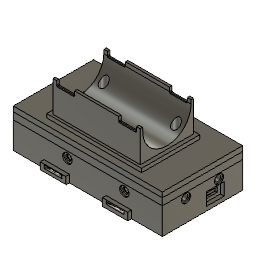
Display (Autodesk Fusion 360 design; units mm, degrees)
Autodesk Fusion 360 part; units mm, degrees
sketch "Sketch1" plane through (0, 0, 0) normal (0, 0, 1) x (1, 0, 0)
  line L0 (20.6, 4.75) -> (97.2, 4.75)
  line L1 (97.2, 4.75) -> (97.2, 56.75)
  line L2 (97.2, 56.75) -> (20.6, 56.75)
  line L3 (20.6, 56.75) -> (20.6, 4.75)
  line L4 (0, 0) -> (117.8, 0)
  line L5 (117.8, 0) -> (117.8, 63.5)
  line L6 (117.8, 63.5) -> (0, 63.5)
  line L7 (0, 63.5) -> (0, 0)
  dimension "d1" = 76.6
  dimension "d2" = 52
  dimension "d4" = 64
  dimension "d5" = 4.75
  dimension "d6" = 20.6
  dimension "d41" = 20.6
  dimension "d47" = 6.75
  constraint horizontal L0
  constraint vertical L1
  constraint horizontal L2
  constraint vertical L3
  constraint horizontal L4
  constraint vertical L5
  constraint horizontal L6
  constraint vertical L7
  constraint coincident L4.start L7.end
  measures "d1" distance of L0.start L0.end
  measures "d2" distance of L0.start L2.end
  measures "d5" distance of L0 L4
  measures "d6" distance of L3 L7
  measures "d41" distance of L1 L5
  measures "d47" distance of L2 L6
extrude "Extrude1" add sketch "Sketch1" along normal blind 1 makes body 1
sketch "Sketch2" plane through (0, 0, 1) normal (0, 0, 1) x (-1, 0, 0)
  line L0 (-20.6, -4.75) -> (-20.6, -56.75)
  line L1 (-20.6, -56.75) -> (-97.2, -56.75)
  line L2 (-97.2, -56.75) -> (-97.2, -4.75)
  line L3 (-97.2, -4.75) -> (-20.6, -4.75)
  line L4 (0, -63.5) -> (0, 0)
  line L5 (0, 0) -> (-117.8, 0)
  line L6 (-117.8, 0) -> (-117.8, -63.5)
  line L7 (-117.8, -63.5) -> (0, -63.5)
  line L8 (-18.6, -58.5) -> (-105.6, -58.5)
  line L9 (-105.6, -58.5) -> (-105.6, -3)
  line L10 (-105.6, -3) -> (-18.6, -3)
  line L11 (-18.6, -3) -> (-18.6, -58.5)
  dimension "d9" = 55.5
  dimension "d14" = 2
  dimension "d15" = 8.4
  dimension "d46" = 1.75
  constraint horizontal L8
  constraint vertical L9
  constraint horizontal L10
  constraint vertical L11
  measures "d9" distance of L8.start L10.end
  measures "d14" distance of L0 L11
  measures "d15" distance of L2 L9
  measures "d46" distance of L1 L8
extrude "Extrude2" add sketch "Sketch2" along normal blind 4.56 contours L4 L5 L6 L7 bodies 1
sketch "Sketch3" plane through (0, 0, 5.56) normal (0, 0, 1) x (-1, 0, 0)
  line L0 (-18.6, -3) -> (-18.6, -58.5)
  line L1 (-18.6, -58.5) -> (-105.6, -58.5)
  line L2 (-105.6, -58.5) -> (-105.6, -3)
  line L3 (-117.8, -63.5) -> (0, -63.5)
  line L4 (0, -63.5) -> (0, 0)
  line L5 (0, 0) -> (-117.8, 0)
  line L6 (-117.8, 0) -> (-117.8, -63.5)
  line L7 (-11, -50.1) -> (-18.1, -50.1)
  line L8 (-18.1, -50.1) -> (-18.1, -43.1)
  line L9 (-18.1, -43.1) -> (-11, -43.1)
  line L10 (-11, -43.1) -> (-11, -50.1)
  circle A0 centre (-14.3, -54.9) radius 1.35
  line L11 (-9.2, -61.5) -> (-113, -61.5)
  line L12 (-113, -2) -> (-9.2, -2)
  line L13 (-9.2, -2) -> (-9.2, -61.5)
  line L14 (-105.6, -3) -> (-18.6, -3)
  circle A1 centre (-14.5, -6.6) radius 1.35
  line L15 (-14.5, -66.6204) -> (-14.5, 2.7727) construction
  line L16 (4.0638, -54.9) -> (-136.0957, -54.9) construction
  line L17 (6.1694, -6.6) -> (-139.7576, -6.6) construction
  circle A2 centre (-109.1, -54.9) radius 1.35
  circle A3 centre (-109.1, -6.6) radius 1.35
  line L18 (-109.1, -67.6336) -> (-109.1, 4.2174) construction
  line L19 (-113, -15) -> (-115.8, -15)
  line L20 (-115.8, -15) -> (-115.8, -23)
  line L21 (-115.8, -23) -> (-113, -23)
  line L22 (-113, -23) -> (-113, -15)
  line L23 (-113, -61.5) -> (-113, -23)
  line L24 (-113, -15) -> (-113, -2)
  dimension "d19" = 7
  dimension "d20" = 2.7
  dimension "d24" = 3
  dimension "d25" = 1
  dimension "d26" = 0.5
  dimension "d27" = 1.8
  dimension "d29" = 8.4
  dimension "d30" = 3.6
  dimension "d31" = 4.3
  dimension "d32" = 2.7
  dimension "d33" = 3.6
  dimension "d34" = 4.1
  dimension "d35" = 7.4
  dimension "d36" = 9.4
  dimension "d37" = 2.7
  dimension "d39" = 2.7
  dimension "d40" = 3.5
  dimension "d134" = 8
  dimension "d135" = 2.8
  dimension "d136" = 13
  dimension "d172" = 103.8
  constraint horizontal L7
  constraint vertical L8
  constraint horizontal L9
  constraint vertical L10
  constraint horizontal L11
  constraint vertical L23
  constraint horizontal L12
  constraint vertical L13
  constraint perpendicular L5 L15
  constraint coincident A1.centre L15
  constraint perpendicular L6 L16
  constraint perpendicular L4 L17
  constraint coincident A1.centre L17
  constraint coincident A0.centre L16
  constraint coincident L17 A3.centre
  constraint perpendicular L5 L18
  constraint coincident A3.centre L18
  constraint coincident A2.centre L18
  constraint horizontal L19
  constraint vertical L20
  constraint horizontal L21
  constraint vertical L22
  constraint collinear L22 L24
  constraint collinear L23 L24
  constraint coincident L16 A2.centre
  measures "d19" distance of L7.start L9.end
  measures "d20" diameter of A0
  measures "d24" distance of L1 L11
  measures "d25" distance of L12 L14
  measures "d26" distance of L0 L8
  measures "d27" distance of L10 L13
  measures "d29" distance of L1 L7
  measures "d30" distance of L1 A0.centre
  measures "d31" distance of L0 A0.centre
  measures "d32" diameter of A1
  measures "d33" distance of L14 A1.centre
  measures "d34" distance of L0 A1.centre
  measures "d35" distance of L2 L23
  measures "d36" distance of L0 L13
  measures "d37" diameter of A2
  measures "d39" diameter of A3
  measures "d40" distance of L2 L18
  measures "d134" distance of L19.end L20.end
  measures "d135" distance of L20.end L21.end
  measures "d136" distance of L12 L19
  measures "d172" distance of L11.start L11.end
extrude "Extrude3" add sketch "Sketch3" along normal blind 15.5 contours L3 L4 L5 L6 | L19 L20 L21 L22 bodies 1
extrude "Extrude4" cut sketch "Sketch3" against normal blind 4.96 contours L7 L8 L9 L10 bodies 1
extrude "Extrude5" add sketch "Sketch3" along normal blind 1.5 contours A0 | A1 | A2 | A3 bodies 1
sketch "Sketch4" plane through (0, 0, 21.06) normal (0, 0, 1) x (-1, 0, 0)
  line L0 (-117.8, 0) -> (-117.8, -63.5)
  line L1 (-117.8, -63.5) -> (0, -63.5)
  line L2 (0, -63.5) -> (0, 0)
  line L3 (0, 0) -> (-117.8, 0)
  line L4 (0, 0) -> (-117.8, 0)
  line L5 (-117.8, 0) -> (-117.8, -63.5)
  line L6 (-117.8, -63.5) -> (0, -63.5)
  line L7 (0, -63.5) -> (0, 0)
  circle A0 centre (-14.5, -54.9) radius 2.5
  circle A1 centre (-14.5, -6.6) radius 2.5
  circle A2 centre (-109.1, -54.9) radius 2.5
  circle A3 centre (-109.1, -6.6) radius 2.5
  line L8 (-9.7, -61) -> (-112.5, -61)
  line L9 (-112.5, -61) -> (-112.5, -2.5)
  line L10 (-112.5, -2.5) -> (-9.7, -2.5)
  line L11 (-9.7, -2.5) -> (-9.7, -61)
  line L12 (-14.5, -67.6729) -> (-14.5, 3.504) construction
  line L13 (6.1552, -6.6) -> (-123.4587, -6.6) construction
  line L14 (5.0248, -54.9) -> (-119.1474, -54.9) construction
  line L15 (-109.1, -66.7497) -> (-109.1, 4.6118) construction
  line L16 (-113, -61.5) -> (-113, -2)
  line L17 (-113, -2) -> (-9.2, -2)
  line L18 (-9.2, -2) -> (-9.2, -61.5)
  line L19 (-9.2, -61.5) -> (-113, -61.5)
  line L20 (4.0638, -54.9) -> (-136.0957, -54.9)
  line L21 (-14.5, -66.6204) -> (-14.5, 2.7727)
  line L22 (-109.1, -67.6336) -> (-109.1, 4.2174)
  line L23 (6.1694, -6.6) -> (-139.7576, -6.6)
  line L24 (-9.2, -61.5) -> (-113, -61.5)
  line L25 (-9.2, -2) -> (-9.2, -61.5)
  line L26 (-113, -61.5) -> (-113, -23)
  line L27 (-113, -2) -> (-9.2, -2)
  dimension "d50" = 5
  dimension "d51" = 5
  dimension "d52" = 5
  dimension "d53" = 5
  dimension "d173" = 0.5
  dimension "d174" = 0.5
  dimension "d175" = 0.5
  dimension "d176" = 0.5
  constraint horizontal L4
  constraint vertical L5
  constraint horizontal L6
  constraint vertical L7
  constraint coincident L0.end L1.start
  constraint coincident L2.end L3.start
  constraint horizontal L8
  constraint vertical L9
  constraint horizontal L10
  constraint vertical L11
  constraint perpendicular L7 L13
  constraint perpendicular L4 L15
  constraint collinear L14 L20
  constraint collinear L12 L21
  constraint collinear L15 L22
  constraint collinear L13 L23
  constraint coincident A1.centre L13
  constraint coincident A1.centre L12
  constraint coincident A0.centre L12
  constraint coincident A0.centre L14
  constraint coincident A2.centre L15
  constraint coincident A2.centre L14
  constraint coincident A3.centre L13
  constraint coincident A3.centre L15
  measures "d50" diameter of A0
  measures "d51" diameter of A1
  measures "d52" diameter of A2
  measures "d53" diameter of A3
  measures "d173" distance of L8 L24
  measures "d174" distance of L11 L25
  measures "d175" distance of L9 L26
  measures "d176" distance of L10 L27
extrude "Extrude6" add sketch "Sketch4" along normal blind 5.5 separate body makes body 2
extrude "Extrude7" add sketch "Sketch4" against normal blind 8.9 contours A2 A3 L9 L20 L22 L23 | A3 L9 L10 L22 L23 | A1 A3 L10 L21 L22 L23 | A2 L8 L9 L20 L22 | A1 L10 L11 L21 L23 | A0 A1 A2 A3 L20 L21 L22 L23 | A0 A2 L8 L20 L21 L22 | A0 A1 L11 L20 L21 L23 | A0 L8 L11 L20 L21 bodies 2
extrude "Extrude8" add sketch "Sketch4" against normal blind 13.9 contours A3 L22 L23 | A3 L22 L23 | A3 L22 L23 | A2 L20 L22 | A2 L20 L22 | A3 L22 L23 | A1 L21 L23 | A1 L21 L23 | A2 L20 L22 | A2 L20 L22 | A1 L21 L23 | A1 L21 L23 | A0 L20 L21 | A0 L20 L21 | A0 L20 L21 | A0 L20 L21 bodies 2
sketch "Sketch5" plane through (0, 0, 0) normal (0, -1, 0) x (1, 0, 0)
  line L0 (0, 0) -> (117.8, 0)
  line L1 (117.8, 0) -> (117.8, 21.06)
  line L2 (117.8, 21.06) -> (0, 21.06)
  line L3 (0, 21.06) -> (0, 0)
  circle A0 centre (87.8, 16.06) radius 3 construction
  line L4 (-16.7106, 16.06) -> (102.3106, 16.06) construction
  circle A1 centre (42.8, 16.06) radius 3 construction
  line L5 (0, 21.06) -> (117.8, 21.06) construction
  dimension "d69" = 6
  dimension "d71" = 30
  dimension "d72" = 6
  dimension "d74" = 5
  dimension "d86" = 45
  constraint perpendicular L3 L4
  constraint coincident A0.centre L4
  constraint midpoint L4 A1.centre
  measures "d69" diameter of A0
  measures "d71" distance of L1 A0.centre
  measures "d72" diameter of A1
  measures "d74" distance of L4 L5
  measures "d86" distance of A0.centre A1.centre
hole "Hole1" at (42.8, 0, 16.06) at (87.8, 0, 16.06) direction (0, 1, 0) diameter 4.5 depth 9 tip angle 180 counterbore diameter 7.5 counterbore depth 1 bodies 1 2
sketch "Sketch9" plane through (0, 63.5, 0) normal (0, 1, 0) x (-1, 0, 0)
  line L0 (-117.8, 0) -> (0, 0)
  line L1 (0, 0) -> (0, 21.06)
  line L2 (0, 21.06) -> (-117.8, 21.06)
  line L3 (-117.8, 21.06) -> (-117.8, 0)
  circle A0 centre (-87.8, 16.06) radius 3 construction
  line L4 (16.7106, 16.06) -> (-102.3106, 16.06) construction
  circle A1 centre (-42.8, 16.06) radius 3 construction
  dimension "d92" = 6
  dimension "d93" = 6
  dimension "d94" = 45
  dimension "d96" = 30
  dimension "d97" = 5
  constraint coincident A0.centre L4
  constraint midpoint A1.centre L4
  measures "d92" diameter of A0
  measures "d93" diameter of A1
  measures "d94" distance of A1.centre A0.centre
  measures "d96" distance of L3 A0.centre
  measures "d97" distance of L2 L4
hole "Hole2" at (87.8, 63.5, 16.06) at (42.8, 63.5, 16.06) direction (0, -1, 0) diameter 4.5 depth 9 tip angle 180 counterbore diameter 7.5 counterbore depth 1 bodies 1 2
sketch "Sketch10" plane through (117.8, 0, 0) normal (1, 0, 0) x (0, 1, 0)
  line L0 (0, 0) -> (63.5, 0)
  line L1 (63.5, 0) -> (63.5, 21.06)
  line L2 (63.5, 21.06) -> (0, 21.06)
  line L3 (0, 21.06) -> (0, 0)
  line L4 (-3.7247, 17.06) -> (70.5896, 17.06) construction
  circle A0 centre (18.75, 17.06) radius 3 construction
  circle A1 centre (44.75, 17.06) radius 3 construction
  line L5 (44.75, 17.06) -> (44.75, 10.4391) construction
  dimension "d103" = 4
  dimension "d104" = 6
  dimension "d105" = 6
  dimension "d106" = 18.75
  dimension "d107" = 18.75
  constraint perpendicular L3 L4
  constraint coincident L4 A0.centre
  constraint coincident L4 A1.centre
  constraint coincident A1.centre L5.start
  constraint perpendicular L4 L5
  measures "d103" distance of L2 L4
  measures "d104" diameter of A0
  measures "d105" diameter of A1
  measures "d106" distance of L3 A0.centre
  measures "d107" distance of L1 A1.centre
hole "Hole3" at (117.8, 18.75, 17.06) at (117.8, 44.75, 17.06) direction (-1, 0, 0) diameter 4.5 depth 9 tip angle 180 counterbore diameter 7.2 counterbore depth 1 bodies 1 2
sketch "Sketch11" plane through (0, 0, 26.56) normal (0, 0, 1) x (-1, 0, 0)
  line L0 (0, -63.5) -> (0, 0)
  line L1 (0, 0) -> (-117.8, 0)
  line L2 (-117.8, 0) -> (-117.8, -63.5)
  line L3 (-117.8, -63.5) -> (0, -63.5)
  line L4 (-5, -71.4838) -> (-5, 10.5389) construction
  circle A0 centre (-5, -45.5) radius 3 construction
  circle A1 centre (-5, -18) radius 3 construction
  dimension "d113" = 6
  dimension "d114" = 6
  dimension "d115" = 18
  dimension "d116" = 18
  dimension "d117" = 5
  constraint perpendicular L3 L4
  constraint coincident L4 A0.centre
  constraint coincident L4 A1.centre
  measures "d113" diameter of A0
  measures "d114" diameter of A1
  measures "d115" distance of L3 A0.centre
  measures "d116" distance of L1 A1.centre
  measures "d117" distance of L0 L4
hole "Hole4" at (5, 45.5, 26.56) at (5, 18, 26.56) direction (0, 0, -1) diameter 4.5 depth 9 tip angle 180 counterbore diameter 7.5 counterbore depth 3 bodies 1 2
sketch "Sketch6" plane through (0, 0, 26.56) normal (0, 0, 1) x (-1, 0, 0)
  line L0 (0, -63.5) -> (0, 0)
  line L1 (0, 0) -> (-117.8, 0)
  line L2 (-117.8, 0) -> (-117.8, -63.5)
  line L3 (-117.8, -63.5) -> (0, -63.5)
  line L4 (-11.3, -60.5) -> (-110.8, -60.5)
  line L5 (-110.8, -60.5) -> (-110.8, -3)
  line L6 (-110.8, -3) -> (-11.3, -3)
  line L7 (-11.3, -3) -> (-11.3, -60.5)
  circle A0 centre (-5, -45.5) radius 3.75
  circle A1 centre (-5, -18) radius 3.75
  line L8 (-117.8, -31.75) -> (0, -31.75) construction
  dimension "d80" = 99.5
  dimension "d81" = 57.5
  dimension "d83" = 7
  dimension "d245" = 28.75
  constraint horizontal L4
  constraint vertical L5
  constraint horizontal L6
  constraint vertical L7
  constraint midpoint L2 L8.start
  constraint midpoint L0 L8.end
  measures "d80" distance of L4.start L4.end
  measures "d81" distance of L4.start L6.end
  measures "d83" distance of L2 L5
  measures "d245" distance of L6 L8
extrude "Extrude9" cut sketch "Sketch6" against normal blind 7 contours L4 L5 L6 L7 bodies 2
sketch "Sketch7" plane through (0, 0, 19.56) normal (0, 0, 1) x (-1, 0, 0)
  line L0 (-11.3, -3) -> (-110.8, -3)
  line L1 (-11.3, -33) -> (-16.3, -33)
  line L2 (-16.3, -33) -> (-16.3, -13)
  line L3 (-16.3, -13) -> (-11.3, -13)
  line L4 (-11.3, -13) -> (-11.3, -33)
  line L5 (-11.3, -3) -> (-11.3, -60.5)
  line L6 (-11.3, -60.5) -> (-11.3, -3)
  line L7 (-110.8, -3) -> (-110.8, -60.5)
  line L8 (-110.8, -60.5) -> (-11.3, -60.5)
  dimension "d87" = 5
  dimension "d88" = 20
  dimension "d91" = 10
  constraint horizontal L1
  constraint vertical L2
  constraint horizontal L3
  constraint vertical L4
  constraint collinear L4 L5
  measures "d87" distance of L1.start L1.end
  measures "d88" distance of L1.end L2.end
  measures "d91" distance of L0 L3
extrude "Extrude10" cut sketch "Sketch7" against normal through all contours L1 L2 L3 L4 L5 L6 bodies 2
sketch "Sketch12" plane through (0, 63.5, 0) normal (0, 1, 0) x (-1, 0, 0)
  line L0 (-117.8, 21.06) -> (0, 21.06)
  line L1 (0, 21.06) -> (0, 26.56)
  line L2 (0, 26.56) -> (-117.8, 26.56)
  line L3 (-117.8, 26.56) -> (-117.8, 21.06)
  line L4 (-22.815, 25.21) -> (-17.185, 25.21)
  line L5 (-15.435, 23.46) -> (-15.435, 23.26)
  line L6 (-17.185, 21.51) -> (-22.815, 21.51)
  line L7 (-24.565, 23.26) -> (-24.565, 23.46)
  arc A0 (-22.815, 25.21) -> (-24.565, 23.46) centre (-22.815, 23.46) ccw
  arc A1 (-24.565, 23.26) -> (-22.815, 21.51) centre (-22.815, 23.26) ccw
  arc A2 (-17.185, 21.51) -> (-15.435, 23.26) centre (-17.185, 23.26) ccw
  arc A3 (-15.435, 23.46) -> (-17.185, 25.21) centre (-17.185, 23.46) ccw
  arc A4 (-15.085, 23.46) -> (-17.185, 25.56) centre (-17.185, 23.46) ccw
  line L8 (-22.815, 25.56) -> (-17.185, 25.56)
  arc A5 (-22.815, 25.56) -> (-24.915, 23.46) centre (-22.815, 23.46) ccw
  line L9 (-24.915, 23.26) -> (-24.915, 23.46)
  arc A6 (-24.915, 23.26) -> (-22.815, 21.16) centre (-22.815, 23.26) ccw
  line L10 (-17.185, 21.16) -> (-22.815, 21.16)
  arc A7 (-17.185, 21.16) -> (-15.085, 23.26) centre (-17.185, 23.26) ccw
  line L11 (-15.085, 23.46) -> (-15.085, 23.26)
  point P0 (-24.565, 25.21)
  point P1 (-15.435, 25.21)
  point P2 (-24.565, 21.51)
  dimension "d123" = 15.435
  dimension "d124" = 9.13
  dimension "d125" = 3.7
  dimension "d126" = 5.5
  dimension "d127" = 1.35
  dimension "d128" = 1.75
  dimension "d131" = -0.35
  constraint horizontal L4
  constraint vertical L5
  constraint horizontal L6
  constraint vertical L7
  constraint coincident P0 L4
  constraint coincident P0 L7
  constraint tangent L4 A0
  constraint tangent L7 A0
  constraint coincident P2 L6
  constraint coincident P2 L7
  constraint tangent L6 A1
  constraint tangent L7 A1
  constraint equal A0 A1
  constraint tangent L5 A2
  constraint tangent L6 A2
  constraint equal A0 A2
  constraint coincident P1 L4
  constraint coincident P1 L5
  constraint tangent L4 A3
  constraint tangent L5 A3
  constraint equal A0 A3
  measures "d123" distance of L1 L5
  measures "d124" distance of P0 P1
  measures "d125" distance of P0 P2
  measures "d126" distance of L0.end L1.end
  measures "d127" distance of L2 L4
  measures "d128" radius of A0
extrude "Extrude11" cut sketch "Sketch12" against normal blind 4 contours L4 L5 L6 L7 A0 A1 A2 A3 bodies 2
extrude "Extrude12" cut sketch "Sketch12" against normal blind 1.17 contours A4 L8 A5 L9 A6 L10 A7 L11 bodies 2
extrude "Extrude13" cut sketch "Sketch3" along normal blind 6 contours L19 L20 L21 L22 bodies 1
sketch "Sketch14" plane through (0, 61.5, 0) normal (0, -1, 0) x (1, 0, 0)
  line L0 (9.2, 5.56) -> (113, 5.56)
  line L1 (113, 5.56) -> (113, 21.06)
  line L2 (113, 21.06) -> (9.2, 21.06)
  line L3 (9.2, 21.06) -> (9.2, 5.56)
  line L4 (55.15, 7.06) -> (71.15, 7.06)
  line L5 (71.15, 7.06) -> (71.15, 9.56)
  line L6 (71.15, 9.56) -> (55.15, 9.56)
  line L7 (55.15, 9.56) -> (55.15, 7.06)
  circle A0 centre (87.8, 16.06) radius 2.25
  circle A1 centre (42.8, 16.06) radius 2.25
  dimension "d139" = 45.95
  dimension "d140" = 1.5
  dimension "d141" = 16
  dimension "d142" = 2.5
  constraint horizontal L4
  constraint vertical L5
  constraint horizontal L6
  constraint vertical L7
  measures "d139" distance of L3 L7
  measures "d140" distance of L0 L4
  measures "d141" distance of L5.end L6.end
  measures "d142" distance of L4.end L5.end
extrude "Extrude14" cut sketch "Sketch14" against normal through all contours L4 L5 L6 L7 bodies 1
sketch "Sketch15" plane through (113, 0, 0) normal (-1, 0, 0) x (0, -1, 0)
  line L0 (-23, 5.56) -> (-23, 11.56)
  line L1 (-23, 11.56) -> (-15, 11.56)
  line L2 (-15, 11.56) -> (-15, 5.56)
  line L3 (-15, 5.56) -> (-2, 5.56)
  line L4 (-2, 5.56) -> (-2, 21.06)
  line L5 (-2, 21.06) -> (-61.5, 21.06)
  line L6 (-61.5, 21.06) -> (-61.5, 5.56)
  line L7 (-61.5, 5.56) -> (-23, 5.56)
  circle A0 centre (-44.75, 17.06) radius 2.25
  circle A1 centre (-18.75, 17.06) radius 2.25
  line L8 (-37.4, 5.76) -> (-46.4, 5.76)
  line L9 (-46.4, 5.76) -> (-46.4, 9.46)
  line L10 (-46.4, 9.46) -> (-37.4, 9.46)
  line L11 (-37.4, 9.46) -> (-37.4, 5.76)
  line L12 (-46.4, 5.76) -> (-46.4, 5.56) construction
  dimension "d144" = 15.1
  dimension "d145" = 9
  dimension "d146" = 3.7
  dimension "d208" = 0.2
  constraint horizontal L8
  constraint vertical L9
  constraint horizontal L10
  constraint vertical L11
  constraint coincident L11 L8.start
  constraint coincident L7 L12.end
  constraint perpendicular L7 L12
  measures "d144" distance of L6 L9
  measures "d145" distance of L9.end L10.end
  measures "d146" distance of L10.end L8.start
  measures "d208" distance of L8.end L12.end
extrude "Extrude15" cut sketch "Sketch15" against normal through all contours L8 L9 L10 L11 bodies 1
sketch "Sketch16" plane through (117.8, 0, 0) normal (1, 0, 0) x (0, 1, 0)
  circle A0 centre (18.75, 17.06) radius 3.6
  line L0 (0, 0) -> (63.5, 0)
  line L1 (63.5, 0) -> (63.5, 21.06)
  line L2 (63.5, 21.06) -> (0, 21.06)
  line L3 (0, 21.06) -> (0, 0)
  line L4 (34.9, 13.31) -> (48.9, 13.31)
  line L5 (48.9, 13.31) -> (48.9, 3.31)
  line L6 (48.9, 3.31) -> (34.9, 3.31)
  line L7 (34.9, 3.31) -> (34.9, 13.31)
  line L8 (41.9, 10.16) -> (41.9, 13.31) construction
  line L9 (37.4, 8.31) -> (34.9, 8.31) construction
  line L10 (37.4, 5.76) -> (37.4, 9.46)
  line L11 (37.4, 9.46) -> (46.4, 9.46)
  line L12 (46.4, 9.46) -> (46.4, 5.76)
  line L13 (46.4, 5.76) -> (37.4, 5.76)
  circle A1 centre (44.75, 17.06) radius 3.6
  dimension "d151" = 14
  dimension "d152" = 10
  constraint horizontal L4
  constraint vertical L5
  constraint horizontal L6
  constraint vertical L7
  constraint midpoint L4 L8.end
  constraint midpoint L7 L9.end
  constraint horizontal L9
  constraint vertical L8
  measures "d151" distance of L4.start L4.end
  measures "d152" distance of L4.start L6.end
extrude "Extrude16" cut sketch "Sketch16" against normal blind 3 contours L4 L5 L6 L7 | L10 L11 L12 L13 bodies 1
sketch "Sketch17" plane through (0, 0, 26.56) normal (0, 0, 1) x (-1, 0, 0)
  line L0 (-110.8, -60.5) -> (-110.8, -3)
  line L1 (-110.8, -3) -> (-11.3, -3)
  line L2 (-11.3, -3) -> (-11.3, -60.5)
  line L3 (-11.3, -60.5) -> (-110.8, -60.5)
  circle A0 centre (-5, -45.5) radius 3.75
  circle A1 centre (-5, -18) radius 3.75
  line L4 (0, -63.5) -> (0, 0)
  line L5 (0, 0) -> (-117.8, 0)
  line L6 (-117.8, 0) -> (-117.8, -63.5)
  line L7 (-117.8, -63.5) -> (0, -63.5)
  line L8 (-117.8, 0) -> (0, 0)
  line L9 (0, 0) -> (0, -63.5)
  line L10 (0, -63.5) -> (-117.8, -63.5)
  line L11 (-117.8, -63.5) -> (-117.8, 0)
  line L12 (-11.8, -60.25) -> (-110.3, -60.25)
  line L13 (-110.3, -60.25) -> (-110.3, -3.25)
  line L14 (-110.3, -3.25) -> (-11.8, -3.25)
  line L15 (-11.8, -3.25) -> (-11.8, -60.25)
  dimension "d156" = 98.5
  dimension "d157" = 57
  dimension "d158" = 7.5
  dimension "d159" = 3.25
  constraint horizontal L8
  constraint vertical L9
  constraint horizontal L10
  constraint vertical L11
  constraint coincident L4.start L7.end
  constraint coincident L5.end L6.start
  constraint perpendicular L12 L13
  constraint perpendicular L12 L15
  measures "d156" distance of L13.end L14.end
  measures "d157" distance of L12.end L13.end
  measures "d158" distance of L11 L13
  measures "d159" distance of L8 L14
extrude "Extrude18" add sketch "Sketch17" along normal blind 4 separate body contours L0 L1 L2 L3 | A0 | A1 | L4 L5 L6 L7 L8 L9 L10 L11 | L12 L13 L14 L15 makes body 3
extrude "Extrude19" add sketch "Sketch17" against normal blind 1 contours L12 L13 L14 L15 bodies 3
sketch "Sketch18" plane through (0, 0, 30.56) normal (0, 0, 1) x (-1, 0, 0)
  line L0 (-117.8, -63.5) -> (0, -63.5)
  line L1 (0, -63.5) -> (0, 0)
  line L2 (0, 0) -> (-117.8, 0)
  line L3 (-117.8, 0) -> (-117.8, -63.5)
  line L4 (-96.4, -5) -> (-21.4, -5)
  line L5 (-21.4, -5) -> (-21.4, -51)
  line L6 (-21.4, -51) -> (-96.4, -51)
  line L7 (-96.4, -51) -> (-96.4, -5)
  line L8 (-58.9, 0) -> (-58.9, -63.5) construction
  line L9 (-117.8, -31.75) -> (0, -31.75) construction
  dimension "d166" = 46
  dimension "d167" = 75
  dimension "d169" = 37.5
  dimension "d177" = 5
  constraint horizontal L4
  constraint vertical L5
  constraint horizontal L6
  constraint vertical L7
  constraint midpoint L2 L8.start
  constraint midpoint L0 L8.end
  constraint midpoint L3 L9.start
  constraint midpoint L1 L9.end
  measures "d166" distance of L4.start L6.end
  measures "d167" distance of L4.start L4.end
  measures "d169" distance of L5 L8
  measures "d177" distance of L2 L4
extrude "Extrude20" add sketch "Sketch18" along normal blind 3 separate body contours L4 L5 L6 L7 makes body 4
sketch "Sketch19" plane through (0, 0, 33.56) normal (0, 0, 1) x (-1, 0, 0)
  line L0 (-96.4, -51) -> (-21.4, -51)
  line L1 (-21.4, -51) -> (-21.4, -5)
  line L2 (-21.4, -5) -> (-96.4, -5)
  line L3 (-96.4, -5) -> (-96.4, -51)
  line L4 (-58.9, -5) -> (-58.9, -51) construction
  line L5 (-93.4, -6.95) -> (-24.4, -6.95)
  line L6 (-24.4, -6.95) -> (-24.4, -49.05)
  line L7 (-24.4, -49.05) -> (-93.4, -49.05)
  line L8 (-93.4, -49.05) -> (-93.4, -6.95)
  line L9 (-21.4, -28) -> (-96.4, -28) construction
  circle A0 centre (-30.4, -14.95) radius 3
  circle A1 centre (-87.4, -14.95) radius 3
  circle A2 centre (-30.4, -41.05) radius 3
  circle A3 centre (-87.4, -41.05) radius 3
  dimension "d181" = 42.1
  dimension "d182" = 34.5
  dimension "d184" = 21.05
  dimension "d234" = 6
  dimension "d237" = 6
  dimension "d238" = 8
  constraint midpoint L2 L4.start
  constraint midpoint L0 L4.end
  constraint horizontal L5
  constraint vertical L6
  constraint horizontal L7
  constraint vertical L8
  constraint midpoint L1 L9.start
  constraint midpoint L3 L9.end
  constraint symmetric L4 A0 A1
  constraint symmetric L9 A0 A2
  constraint symmetric L9 A1 A3
  measures "d181" distance of L5 L7
  measures "d182" distance of L4 L8
  measures "d184" distance of L5 L9
  measures "d234" diameter of A0
  measures "d237" distance of L6 A0.centre
  measures "d238" distance of L5 A0.centre
extrude "Extrude21" add sketch "Sketch19" along normal blind 24.5 contours L5 L6 L7 L8 | A0 | A1 | A2 | A3 bodies 4
sketch "Sketch20" plane through (93.4, 0, 0) normal (1, 0, 0) x (0, 1, 0)
  line L0 (6.95, 33.56) -> (49.05, 33.56)
  line L1 (49.05, 33.56) -> (49.05, 58.06)
  line L2 (49.05, 58.06) -> (6.95, 58.06)
  line L3 (6.95, 58.06) -> (6.95, 33.56)
  line L4 (28, 58.06) -> (28, 33.56) construction
  line L5 (8.95, 55.06) -> (8.95, 58.06)
  line L6 (47.05, 55.06) -> (47.05, 58.06)
  line L7 (8.95, 58.06) -> (47.05, 58.06)
  arc A0 (8.95, 55.06) -> (47.05, 55.06) centre (28, 55.06) ccw
  dimension "d187" = 38.1
  dimension "d227" = 3
  constraint midpoint L2 L4.start
  constraint midpoint L0 L4.end
  constraint coincident A0.centre L4
  constraint tangent L5 A0
  constraint perpendicular L2 L5
  constraint tangent L6 A0
  constraint perpendicular L2 L6
  constraint coincident L2 L5.end
  constraint coincident L2 L6.end
  measures "d187" diameter of A0
  measures "d227" distance of L2 A0.centre
extrude "Extrude22" cut sketch "Sketch20" against normal through all contours L2 L5 L6 L7 A0 bodies 4
sketch "Sketch21" plane through (0, 0, 0) normal (0, 0, -1) x (1, 0, 0)
  line L0 (20.6, -56.75) -> (20.6, -4.75)
  line L1 (20.6, -4.75) -> (97.2, -4.75)
  line L2 (97.2, -4.75) -> (97.2, -56.75)
  line L3 (97.2, -56.75) -> (20.6, -56.75)
  line L4 (0, 0) -> (0, -63.5)
  line L5 (0, -63.5) -> (117.8, -63.5)
  line L6 (117.8, -63.5) -> (117.8, 0)
  line L7 (117.8, 0) -> (0, 0)
  line L8 (24.4, -63.5) -> (44.4, -63.5)
  line L9 (44.4, -63.5) -> (44.4, -66.5)
  line L10 (44.4, -66.5) -> (24.4, -66.5)
  line L11 (24.4, -66.5) -> (24.4, -63.5)
  line L12 (58.9, 0) -> (58.9, -63.5) construction
  line L13 (0, -31.75) -> (117.8, -31.75) construction
  line L14 (73.4, -66.5) -> (93.4, -66.5)
  line L15 (93.4, -66.5) -> (93.4, -63.5)
  line L16 (93.4, -63.5) -> (73.4, -63.5)
  line L17 (73.4, -63.5) -> (73.4, -66.5)
  line L18 (44.4, 3) -> (24.4, 3)
  line L19 (24.4, 3) -> (24.4, 0)
  line L20 (24.4, 0) -> (44.4, 0)
  line L21 (44.4, 0) -> (44.4, 3)
  line L22 (73.4, 3) -> (93.4, 3)
  line L23 (93.4, 3) -> (93.4, 0)
  line L24 (73.4, 0) -> (73.4, 3)
  line L25 (93.4, 0) -> (73.4, 0)
  dimension "d189" = 20
  dimension "d190" = 3
  dimension "d209" = 24.4
  constraint horizontal L8
  constraint vertical L9
  constraint horizontal L10
  constraint vertical L11
  constraint coincident L5 L8.start
  constraint midpoint L7 L12.start
  constraint midpoint L5 L12.end
  constraint midpoint L4 L13.start
  constraint midpoint L6 L13.end
  constraint symmetric L8.start L12 L15.end
  constraint symmetric L8.end L12 L16.end
  constraint symmetric L9.end L12 L14.start
  constraint symmetric L10.end L12 L14.end
  constraint symmetric L8.start L13 L19.end
  constraint symmetric L8.end L13 L20.end
  constraint symmetric L9.end L13 L18.start
  constraint symmetric L10.end L13 L18.end
  constraint symmetric L13 L14.start L22.start
  constraint symmetric L13 L14.end L22.end
  constraint symmetric L13 L15.end L23.end
  constraint symmetric L13 L16.end L24.start
  measures "d189" distance of L8.start L8.end
  measures "d190" distance of L8.start L10.end
  measures "d209" distance of L4 L11
extrude "Extrude23" add sketch "Sketch21" against normal blind 6 contours L7 L18 L19 L20 L21 | L5 L8 L9 L10 L11 | L7 L22 L23 L24 L25 | L5 L14 L15 L16 L17 bodies 1
ref_plane "WorkPlane1" through (27.4, 31.75, 10.53) normal (-1, 0, 0) x (0, -1, 0)
sketch "Sketch22" plane through (27.4, 0, 0) normal (-1, 0, 0) x (0, -1, 0)
  line L0 (-62.5, 0) -> (-60.5, 0)
  line L1 (-66.5, 0) -> (-66.5, 3) construction
  line L2 (-62.5, 0) -> (-66.5, 0) construction
  line L3 (-66.5, 3) -> (-66.5, 5)
  arc A0 (-62.5, 0) -> (-66.5, 3) centre (-67.0981, -1.9641) ccw
  arc A1 (-60.5, 0) -> (-66.5, 5) centre (-67.9698, -2.8638) ccw
  line L4 (3, 0) -> (-66.5, 0) construction
  line L5 (-31.75, 0) -> (-31.75, 8.9717) construction
  arc A2 (3, 5) -> (-3, 0) centre (4.4698, -2.8638) ccw
  line L6 (-1, 0) -> (-3, 0)
  arc A3 (3, 3) -> (-1, 0) centre (3.5981, -1.9641) ccw
  line L7 (3, 3) -> (3, 5)
  dimension "d198" = 2
  dimension "d199" = 2
  dimension "d200" = 4
  dimension "d201" = 3
  dimension "d202" = 8
  dimension "d203" = 5
  dimension "d210" = 69.5
  dimension "d211" = 3
  constraint horizontal L0
  constraint vertical L1
  constraint perpendicular L1 L2
  constraint parallel L1 L3
  constraint horizontal L4
  constraint coincident origin L4
  constraint coincident L1.start L2.end
  constraint midpoint L4 L5.start
  constraint perpendicular L4 L5
  constraint symmetric L0.start L5 L6.start
  constraint symmetric L0.end L5 A2.end
  constraint symmetric L1.end L5 A3.start
  constraint symmetric L3.end L5 A2.start
  constraint symmetric A0 L5 A3
  constraint symmetric A1 L5 A2
  measures "d198" distance of L0.start L0.end
  measures "d199" distance of L1.end L3.end
  measures "d200" distance of L0.start L1.start
  measures "d201" distance of L1.end L1.start
  measures "d202" radius of A1
  measures "d203" radius of A0
  measures "d210" distance of L4.start L1.start
  measures "d211" distance of origin L4.start
extrude "Extrude24" cut sketch "Sketch22" against normal blind 14 bodies 1
fillet "Fillet1" radius 0.5 6 edges at (34.4, 1, 0) (34.4, -3, 0) (34.4, -3, 5) (34.4, 66.5, 5) (34.4, 66.5, 0) (34.4, 62.5, 0) on bodies 1
ref_plane "WorkPlane2" through (90.4, 31.75, 10.53) normal (1, 0, 0) x (0, 1, 0)
sketch "Sketch23" plane through (90.4, 0, 0) normal (1, 0, 0) x (0, 1, 0)
  arc A0 (-60.5, 0) -> (-66.5, 5) centre (-67.9698, -2.8638) ccw
  line L0 (-62.5, 0) -> (-60.5, 0)
  arc A1 (-62.5, 0) -> (-66.5, 3) centre (-67.0981, -1.9641) ccw
  line L1 (-66.5, 3) -> (-66.5, 5)
  line L2 (-3, 0) -> (66.5, 0) construction
  line L3 (3, 0) -> (1, 0)
  line L4 (-3, 3) -> (-3, 5)
  arc A2 (3, 0) -> (-3, 5) centre (-4.4698, -2.8638) ccw
  arc A3 (1, 0) -> (-3, 3) centre (-3.5981, -1.9641) ccw
  line L5 (-3, 0) -> (-3, 3) construction
  line L6 (31.75, 0) -> (31.75, 8.7682) construction
  line L7 (66.5, 3) -> (66.5, 5)
  arc A4 (66.5, 3) -> (62.5, 0) centre (67.0981, -1.9641) ccw
  line L8 (60.5, 0) -> (62.5, 0)
  arc A5 (66.5, 5) -> (60.5, 0) centre (67.9698, -2.8638) ccw
  dimension "d213" = 2
  dimension "d214" = 2
  dimension "d215" = 8
  dimension "d216" = 5
  dimension "d217" = 69.5
  dimension "d218" = 3
  dimension "d219" = 4
  dimension "d220" = 2
  dimension "d221" = 2
  dimension "d222" = 3
  dimension "d223" = 5
  dimension "d224" = 8
  constraint horizontal L0
  constraint horizontal L2
  constraint coincident origin L2
  constraint coincident L2 L3.start
  constraint coincident L2 L3.end
  constraint perpendicular L2 L4
  constraint perpendicular L2 L5
  constraint coincident L4.start A3.end
  constraint midpoint L2 L6.start
  constraint perpendicular L2 L6
  constraint symmetric L3.start L6 L8.start
  constraint symmetric L3.end L6 A4.end
  constraint symmetric L4.start L6 L7.start
  constraint symmetric L4.end L6 L7.end
  constraint symmetric A2 L6 A5
  constraint symmetric A3 L6 A4
  measures "d213" distance of A0.start L0.start
  measures "d214" distance of A1.end A0.end
  measures "d215" radius of A0
  measures "d216" radius of A1
  measures "d217" distance of L2.start L2.end
  measures "d218" distance of origin L2.start
  measures "d219" distance of L2.start L3.end
  measures "d220" distance of L3.start L3.end
  measures "d221" distance of L4.start L4.end
  measures "d222" distance of L2.start L4.start
  measures "d223" radius of A3
  measures "d224" radius of A2
extrude "Extrude25" cut sketch "Sketch23" against normal blind 14 contours L3 L4 A2 A3 | L7 A4 L8 A5 bodies 1
sketch "Sketch24" plane through (0, 6.95, 0) normal (0, -1, 0) x (1, 0, 0)
  line L0 (24.4, 33.56) -> (93.4, 33.56)
  line L1 (93.4, 33.56) -> (93.4, 58.06)
  line L2 (93.4, 58.06) -> (24.4, 58.06)
  line L3 (24.4, 58.06) -> (24.4, 33.56)
  line L4 (27.4, 58.06) -> (41.4, 58.06)
  line L5 (41.4, 58.06) -> (41.4, 54.5036)
  line L6 (41.4, 54.5036) -> (27.4, 54.5036)
  line L7 (27.4, 54.5036) -> (27.4, 58.06)
  line L8 (58.9, 58.06) -> (58.9, 47.5566) construction
  line L9 (76.4, 54.5036) -> (90.4, 54.5036)
  line L10 (90.4, 54.5036) -> (90.4, 58.06)
  line L11 (90.4, 58.06) -> (76.4, 58.06)
  line L12 (76.4, 58.06) -> (76.4, 54.5036)
  dimension "d228" = 3
  dimension "d229" = 14
  constraint horizontal L4
  constraint vertical L5
  constraint horizontal L6
  constraint vertical L7
  constraint coincident L2 L4.start
  constraint midpoint L2 L8.start
  constraint perpendicular L2 L8
  constraint symmetric L4.start L8 L10.end
  constraint symmetric L4.end L8 L11.end
  constraint symmetric L5.end L8 L9.start
  constraint symmetric L6.end L8 L9.end
  measures "d228" distance of L3 L7
  measures "d229" distance of L5.end L6.end
extrude "Extrude26" cut sketch "Sketch24" against normal through all contours L2 L4 L5 L6 L7 | L2 L9 L10 L11 L12 bodies 4
fillet "Fillet2" radius 0.5 16 edges at (27.4, 7.9541, 54.5036) (34.4, 6.95, 54.5036) (34.4, 8.9581, 54.5036) (41.4, 7.9541, 54.5036) (90.4, 7.9541, 54.5036) (83.4, 8.9581, 54.5036) (83.4, 6.95, 54.5036) (76.4, 7.9541, 54.5036) (76.4, 48.0459, 54.5036) (83.4, 47.0419, 54.5036) (83.4, 49.05, 54.5036) (90.4, 48.0459, 54.5036) (41.4, 48.0459, 54.5036) (34.4, 49.05, 54.5036) (34.4, 47.0419, 54.5036) (27.4, 48.0459, 54.5036) on bodies 4
hole "Hole5" at (30.4, 14.95, 33.56) at (30.4, 41.05, 33.56) at (87.4, 41.05, 33.56) at (87.4, 14.95, 33.56) direction (0, 0, -1) diameter 3.5 depth 10 tip angle 180 counterbore diameter 5.5 counterbore depth 1 bodies 3 4
extrude "Extrude27" cut sketch "Sketch19" along normal through all contours A0 | A1 | A2 | A3 bodies 4
equation "d5 = 3.7 mm + 2 mm - 0.95 mm"
equation "d6 = d41"
equation "d20 = d37"
equation "d31 = 3.8 mm + 0.3 mm + 0.2 mm"
equation "d32 = d37"
equation "d33 = d30"
equation "d39 = d37"
equation "d40 = 3.2 mm + 0.3 mm"
equation "d47 = 7.25 mm - 0.5 mm"
equation "d81 = 58 mm - 0.5 mm"
equation "d106 = d107"
equation "d123 = 6.7 mm + 4.26 mm - 0.125 mm + 5.6 mm + 1 mm - 2 mm"
equation "d139 = 44.6 mm + 1.35 mm"
equation "d169 = d167 / 2"
equation "d181 = 1.5 in + 4 mm"
equation "d184 = d181 / 2"
equation "d245 = d81 / 2"
named bodies: "display_Body", "display_Cover", "display_BackCover", "display_WheelHolder"
